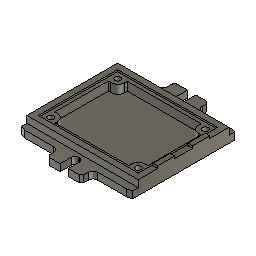
baseplate (Autodesk Fusion 360 design; units mm, degrees)
Autodesk Fusion 360 part; units mm, degrees
sketch "Skizze1" plane through (0, 0, 0) normal (0, 0, 1) x (1, 0, 0)
  line L0 (24.25, 19.75) -> (-24.25, 19.75)
  line L1 (-24.25, 19.75) -> (-24.25, -19.75)
  line L2 (-24.25, -19.75) -> (24.25, -19.75)
  line L3 (24.25, -19.75) -> (24.25, 19.75)
  line L4 (24.25, 19.75) -> (-24.25, -19.75) construction
  line L5 (-24.25, 19.75) -> (24.25, -19.75) construction
  dimension "d1" = 48.5
  dimension "d2" = 39.5
  constraint horizontal L0
  constraint perpendicular L0 L1
  constraint parallel L0 L2
  constraint parallel L1 L3
  constraint coincident L4 origin
  constraint coincident L5 origin
  measures "d1" distance of L1.end L2.end
  measures "d2" distance of L0.end L1.end
extrude "Extrusion1" add sketch "Skizze1" along normal blind 6
sketch "Skizze2" plane through (0, 0, 6) normal (0, 0, 1) x (-1, 0, 0)
  line L0 (-24.25, 19.75) -> (-24.25, -19.75)
  line L1 (-24.25, -19.75) -> (24.25, -19.75)
  line L2 (24.25, -19.75) -> (24.25, 19.75)
  line L3 (24.25, 19.75) -> (-24.25, 19.75)
  line L4 (-21.75, 17.25) -> (21.75, 17.25)
  line L5 (21.75, 17.25) -> (21.75, -17.25)
  line L6 (21.75, -17.25) -> (-21.75, -17.25)
  line L7 (-21.75, -17.25) -> (-21.75, 17.25)
  line L8 (-21.75, 17.25) -> (21.75, -17.25) construction
  line L9 (21.75, 17.25) -> (-21.75, -17.25) construction
  dimension "d5" = 34.5
  dimension "d6" = 43.5
  constraint horizontal L4
  constraint perpendicular L4 L5
  constraint parallel L4 L6
  constraint parallel L5 L7
  constraint coincident L8 origin
  constraint coincident L9 origin
  measures "d5" distance of L4.end L5.end
  measures "d6" distance of L5.end L6.end
extrude "Extrusion2" cut sketch "Skizze2" against normal blind 0.75 contours L4 L5 L6 L7
sketch "Skizze3" plane through (0, 0, 5.25) normal (0, 0, 1) x (-1, 0, 0)
  line L0 (-21.75, -17.25) -> (21.75, -17.25)
  line L1 (21.75, -17.25) -> (21.75, 17.25)
  line L2 (21.75, 17.25) -> (-21.75, 17.25)
  line L3 (-21.75, 17.25) -> (-21.75, -17.25)
  line L4 (-20.25, -15.75) -> (20.25, -15.75)
  line L5 (20.25, -15.75) -> (20.25, 15.75)
  line L6 (20.25, 15.75) -> (-20.25, 15.75)
  line L7 (-20.25, 15.75) -> (-20.25, -15.75)
  line L8 (-20.25, -15.75) -> (20.25, 15.75) construction
  line L9 (20.25, -15.75) -> (-20.25, 15.75) construction
  dimension "d9" = 1.5
  dimension "d10" = 1.5
  constraint horizontal L4
  constraint perpendicular L4 L5
  constraint parallel L4 L6
  constraint parallel L5 L7
  constraint coincident L8 origin
  constraint coincident L9 origin
  measures "d9" distance of L1 L5
  measures "d10" distance of L0 L4
extrude "Extrusion3" cut sketch "Skizze3" against normal up to surface (3.75 mm away) contours L4 L5 L6 L7
sketch "Skizze4" plane through (0, 0, 1.5) normal (0, 0, 1) x (-1, 0, 0)
  line L0 (-20.25, -15.75) -> (20.25, -15.75)
  line L1 (20.25, -15.75) -> (20.25, 15.75)
  line L2 (20.25, 15.75) -> (-20.25, 15.75)
  line L3 (-20.25, 15.75) -> (-20.25, -15.75)
  line L4 (20.25, -15.75) -> (16.05, -15.75)
  line L5 (16.05, -15.75) -> (16.05, -14.605)
  line L6 (19.05, -11.605) -> (20.25, -11.605)
  line L7 (20.25, -11.605) -> (20.25, -15.75)
  line L8 (20.25, 15.75) -> (16.05, 15.75)
  line L9 (16.05, 15.75) -> (16.05, 14.605)
  line L10 (19.05, 11.605) -> (20.25, 11.605)
  line L11 (20.25, 11.605) -> (20.25, 15.75)
  line L12 (-20.25, -15.75) -> (-16.05, -15.75)
  line L13 (-16.05, -15.75) -> (-16.05, -14.605)
  line L14 (-19.05, -11.605) -> (-20.25, -11.605)
  line L15 (-20.25, -11.605) -> (-20.25, -15.75)
  line L16 (-20.25, 15.75) -> (-16.05, 15.75)
  line L17 (-16.05, 15.75) -> (-16.05, 14.605)
  line L18 (-19.05, 11.605) -> (-20.25, 11.605)
  line L19 (-20.25, 11.605) -> (-20.25, 15.75)
  arc A0 (19.05, -11.605) -> (16.05, -14.605) centre (19.05, -14.605) ccw
  arc A1 (-16.05, -14.605) -> (-19.05, -11.605) centre (-19.05, -14.605) ccw
  arc A2 (-19.05, 11.605) -> (-16.05, 14.605) centre (-19.05, 14.605) ccw
  arc A3 (16.05, 14.605) -> (19.05, 11.605) centre (19.05, 14.605) ccw
  dimension "d13" = 3
  dimension "d15" = 29.21
  dimension "d16" = 38.1
  constraint horizontal L4
  constraint vertical L5
  constraint horizontal L6
  constraint vertical L7
  constraint coincident L0.end L1.start
  constraint horizontal L8
  constraint vertical L9
  constraint horizontal L10
  constraint vertical L11
  constraint coincident L1.end L2.start
  constraint horizontal L12
  constraint vertical L13
  constraint horizontal L14
  constraint vertical L15
  constraint coincident L0.start L3.end
  constraint horizontal L16
  constraint vertical L17
  constraint horizontal L18
  constraint vertical L19
  constraint coincident L2.end L3.start
  constraint collinear L13 L17
  constraint collinear L5 L9
  constraint collinear L6 L14
  constraint collinear L10 L18
  constraint tangent L6 A0
  constraint tangent L5 A0
  constraint tangent L13 A1
  constraint tangent L14 A1
  constraint tangent L17 A2
  constraint tangent L18 A2
  constraint equal A1 A2
  constraint tangent L9 A3
  constraint tangent L10 A3
  constraint equal A1 A3
  constraint equal A0 A1
  constraint equal L5 L9
  constraint equal L6 L14
  measures "d13" radius of A0
  measures "d15" distance of A0.centre A3.centre
  measures "d16" distance of A0.centre A1.centre
extrude "Extrusion4" add sketch "Skizze4" along normal up to surface (3.75 mm away) contours L0 L3 L12 L13 L14 L15 A1 | L0 L1 L4 L5 L6 L7 A0 | L2 L3 L16 L17 L18 L19 A2 | L1 L2 L8 L9 L10 L11 A3
sketch "Skizze5" plane through (0, 0, 5.25) normal (0, 0, 1) x (-1, 0, 0)
  line L0 (-16.05, 15.75) -> (16.05, 15.75)
  line L1 (20.25, 11.605) -> (20.25, -11.605)
  line L2 (16.05, -15.75) -> (-16.05, -15.75)
  line L3 (-20.25, -11.605) -> (-20.25, 11.605)
  line L4 (-21.75, -17.25) -> (21.75, -17.25)
  line L5 (21.75, -17.25) -> (21.75, 17.25)
  line L6 (21.75, 17.25) -> (-21.75, 17.25)
  line L7 (-21.75, 17.25) -> (-21.75, -17.25)
  circle A0 centre (19.05, 14.605) radius 1.25
  line L8 (16.05, 15.75) -> (16.05, 14.605)
  arc A1 (16.05, 14.605) -> (19.05, 11.605) centre (19.05, 14.605) ccw
  line L9 (19.05, 11.605) -> (20.25, 11.605)
  line L10 (20.25, -11.605) -> (19.05, -11.605)
  arc A2 (19.05, -11.605) -> (16.05, -14.605) centre (19.05, -14.605) ccw
  line L11 (16.05, -14.605) -> (16.05, -15.75)
  line L12 (-16.05, -15.75) -> (-16.05, -14.605)
  arc A3 (-16.05, -14.605) -> (-19.05, -11.605) centre (-19.05, -14.605) ccw
  line L13 (-19.05, -11.605) -> (-20.25, -11.605)
  line L14 (-20.25, 11.605) -> (-19.05, 11.605)
  arc A4 (-19.05, 11.605) -> (-16.05, 14.605) centre (-19.05, 14.605) ccw
  line L15 (-16.05, 14.605) -> (-16.05, 15.75)
  dimension "d19" = 2.5
  constraint concentric A0 A1
  measures "d19" diameter of A0
extrude "Extrusion5" cut sketch "Skizze5" against normal through all contours A0
sketch "Skizze6" plane through (0, 0, 0) normal (0, 0, -1) x (1, 0, 0)
  line L0 (24.25, -19.75) -> (24.25, 19.75)
  line L1 (24.25, 19.75) -> (-24.25, 19.75)
  line L2 (-24.25, 19.75) -> (-24.25, -19.75)
  line L3 (-24.25, -19.75) -> (24.25, -19.75)
  line L4 (-19.05, 12.1801) -> (-16.95, 13.3926)
  line L5 (-16.95, 13.3926) -> (-16.95, 15.8174)
  line L6 (-16.95, 15.8174) -> (-19.05, 17.0299)
  line L7 (-19.05, 17.0299) -> (-21.15, 15.8174)
  line L8 (-21.15, 15.8174) -> (-21.15, 13.3926)
  line L9 (-21.15, 13.3926) -> (-19.05, 12.1801)
  circle A0 centre (-19.05, 14.605) radius 1.25
  point P0 (-19.05, 14.605)
  dimension "d21" = 2.1
  constraint vertical L8
  constraint coincident P0 A0.centre
  measures "d21" distance of P0 L9
extrude "Extrusion6" cut sketch "Skizze6" against normal blind 2.2 contours L4 L5 L6 L7 L8 L9 | A0
mirror "Spiegeln1" about plane through (0, 0, 0) normal (1, 0, 0) of "Extrusion5", "Extrusion6"
mirror "Spiegeln2" about plane through (0, 0, 0) normal (0, 1, 0) of "Extrusion5", "Extrusion6", "Spiegeln1"
sketch "Skizze7" plane through (0, -19.75, 0) normal (0, -1, 0) x (1, 0, 0)
  line L0 (-24.25, 0) -> (7.5, 0)
  line L1 (24.25, 0) -> (24.25, 6)
  line L2 (24.25, 6) -> (-24.25, 6)
  line L3 (-24.25, 6) -> (-24.25, 0)
  line L4 (-7.5, 3) -> (7.5, 3)
  line L5 (7.5, 3) -> (7.5, 0)
  line L6 (-7.5, 0) -> (-7.5, 3)
  line L7 (-7.5, 0) -> (7.5, 0)
  line L8 (-24.25, 0) -> (24.25, 0)
  dimension "d26" = 3
  dimension "d44" = 15
  constraint horizontal L4
  constraint vertical L5
  constraint vertical L6
  constraint perpendicular L5 L7
  constraint midpoint L7 L8
  measures "d26" distance of L4.start L6.start
  measures "d44" distance of L4.start L4.end
extrude "Extrusion7" add sketch "Skizze7" along normal blind 8 contours L0 L4 L5 L6 L7 L8
sketch "Skizze10" plane through (0, -19.75, 0) normal (0, -1, 0) x (1, 0, 0)
  line L0 (7.5, 3) -> (7.5, 0)
  line L1 (7.5, 0) -> (24.25, 0)
  line L2 (24.25, 0) -> (24.25, 6)
  line L3 (24.25, 6) -> (-24.25, 6)
  line L4 (-24.25, 6) -> (-24.25, 0)
  line L5 (-24.25, 0) -> (-7.5, 0)
  line L6 (-7.5, 0) -> (-7.5, 3)
  line L7 (-7.5, 3) -> (7.5, 3)
  line L8 (24.25, 3) -> (-24.25, 3)
  constraint midpoint L2 L8.start
  constraint midpoint L4 L8.end
extrude "Extrusion10" add sketch "Skizze10" along normal blind 3 contours L0 L1 L2 L8 | L4 L5 L6 L8
sketch "Skizze8" plane through (0, 0, 3) normal (0, 0, 1) x (-1, 0, 0)
  line L0 (-24.25, 19.75) -> (24.25, 19.75)
  line L1 (24.25, 19.75) -> (24.25, 22.75)
  line L2 (7.5, 27.75) -> (-7.5, 27.75)
  line L3 (-7.5, 27.75) -> (-7.5, 22.75)
  line L4 (-1.8, 27.75) -> (1.8, 27.75)
  line L5 (1.8, 27.75) -> (1.8, 23)
  line L6 (0.1, 21.3) -> (-0.1, 21.3)
  line L7 (-1.8, 23) -> (-1.8, 27.75)
  line L8 (-1.8, 27.75) -> (1.8, 21.3) construction
  line L9 (1.8, 27.75) -> (-1.8, 21.3) construction
  arc A0 (0.1, 21.3) -> (1.8, 23) centre (0.1, 23) ccw
  arc A1 (-1.8, 23) -> (-0.1, 21.3) centre (-0.1, 23) ccw
  line L10 (0, 0) -> (0, 21.3) construction
  line L11 (24.25, 22.75) -> (7.5, 22.75)
  line L12 (7.5, 22.75) -> (7.5, 27.75)
  line L13 (-7.5, 22.75) -> (-24.25, 22.75)
  line L14 (-24.25, 22.75) -> (-24.25, 19.75)
  point P0 (0, 24.525)
  dimension "d30" = 3.6
  dimension "d31" = 1.7
  dimension "d34" = 23
  constraint horizontal L4
  constraint perpendicular L4 L5
  constraint parallel L4 L6
  constraint parallel L5 L7
  constraint coincident L2 L4.start
  constraint coincident L8 P0
  constraint coincident L9 P0
  constraint coincident L8.end L5
  constraint coincident L8.end L6
  constraint tangent L5 A0
  constraint tangent L6 A0
  constraint coincident L9.end L6
  constraint coincident L9.end L7
  constraint tangent L6 A1
  constraint tangent L7 A1
  constraint equal A0 A1
  constraint coincident L10.start origin
  constraint midpoint L6 L10.end
  constraint vertical L10
  measures "d30" distance of L4.start L4.end
  measures "d31" radius of A0
  measures "d34" vertical distance of L10.start A1.centre
extrude "Extrusion8" cut sketch "Skizze8" against normal through all contours L2 L4 L5 L6 L7 A0 A1
mirror "Spiegeln6" about plane through (0, 0, 0) normal (0, 1, 0) of "Extrusion7", "Extrusion8"
sketch "Skizze9" plane through (0, 0, 6) normal (0, 0, 1) x (-1, 0, 0)
  line L0 (21.75, 17.25) -> (21.75, -17.25)
  line L1 (21.75, -17.25) -> (-21.75, -17.25)
  line L2 (-21.75, -17.25) -> (-21.75, 17.25)
  line L3 (-21.75, 17.25) -> (21.75, 17.25)
  line L4 (-24.25, 19.75) -> (-24.25, -19.75)
  line L5 (-24.25, -19.75) -> (24.25, -19.75)
  line L6 (24.25, -19.75) -> (24.25, 19.75)
  line L7 (24.25, 19.75) -> (-24.25, 19.75)
  line L8 (-24.25, 11.37) -> (-22.25, 11.37)
  line L9 (-22.25, 11.37) -> (-22.25, 3.87)
  line L10 (-22.25, 3.87) -> (-24.25, 3.87)
  line L11 (-24.25, 3.87) -> (-24.25, 11.37)
  point P0 (-22.25, 7.62)
  point P1 (-29, 6)
  dimension "d39" = 7.5
  dimension "d43" = 7.62
  dimension "d48" = 0.5
  constraint horizontal L8
  constraint vertical L9
  constraint horizontal L10
  constraint vertical L11
  constraint coincident L4 L8.start
  constraint midpoint L9 P0
  measures "d39" distance of L8.start L10.end
  measures "d43" vertical distance of origin P0
  measures "d48" distance of L2 L9
extrude "Extrusion9" add sketch "Skizze9" along normal blind 1 contours L4 L8 L9 L10 L11
mirror "Spiegeln5" about plane through (0, 0, 0) normal (0, 1, 0) of "Extrusion10", "Extrusion9"
fillet "Abrundung1" radius 2 4 edges at (7.5, -22.75, 1.5) (-7.5, -22.75, 1.5) (7.5, 22.75, 1.5) (-7.5, 22.75, 1.5)
chamfer "Fase2" distance 2 distance2 0.5 2 edges at (-24.25, -22.75, 1.5) (24.25, -22.75, 1.5) measured on face at (-19.3333, -22.75, 1) measured on face at (14.4167, -22.75, 2)
chamfer "Fase3" distance 0.5 distance2 2 2 edges at (24.25, 22.75, 1.5) (-24.25, 22.75, 1.5) measured on face at (24.25, 1.4567, 2) measured on face at (-24.25, 6.75, 1)
chamfer "Fase4" distance 1 distance2 1 4 edges at (7.5, -27.75, 1.5) (-7.5, -27.75, 1.5) (-7.5, 27.75, 1.5) (7.5, 27.75, 1.5) measured on face at (5.6, -27.75, 1) measured on face at (-5.6, -27.75, 2) measured on face at (-7.5, 25.75, 1) measured on face at (7.5, 25.75, 2)
equation "d1 = 43.5 mm + 5 mm"
equation "d2 = 34.5 mm + 5 mm"
equation "d43 = ( 15.24 / 2 ) * 1 mm"
